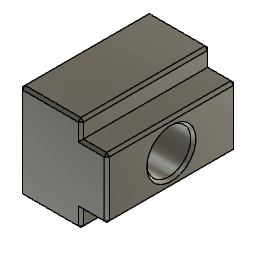
T-Nut_v0.1 (Autodesk Fusion 360 design; units mm, degrees)
Autodesk Fusion 360 part; units mm, degrees
sketch "Sketch1" plane through (0, 0, 0) normal (0, 1, 0) x (1, 0, 0)
  line L0 (-18.22, -14.04) -> (0, -14.04)
  line L1 (0, -14.04) -> (0, 14.04)
  line L2 (0, 14.04) -> (-18.22, 14.04)
  line L3 (-18.22, 14.04) -> (-18.22, -14.04)
  line L4 (0, -5.075) -> (-4, -5.075)
  line L5 (-4, -5.075) -> (-4, -7.75)
  line L6 (-4, -7.75) -> (-14.22, -7.75)
  line L7 (0, 5.075) -> (-4, 5.075)
  line L8 (-4, 5.075) -> (-4, 7.75)
  line L9 (-4, 7.75) -> (-14.22, 7.75)
  line L10 (-14.22, 7.75) -> (-14.22, -7.75)
  line L11 (-18.22, 0) -> (0, 0) construction
  line L12 (-4, -5.075) -> (-4, 5.075) construction
  point P0 (-14.22, 0)
  point P1 (-4, 0)
  dimension "d1" = 28.08
  dimension "d2" = 10.15
  dimension "d3" = 4
  dimension "d4" = 10.22
  dimension "d5" = 15.5
  dimension "d6" = 2.675
  dimension "d7" = 14.22
  dimension "d10" = 4
  constraint horizontal L0
  constraint vertical L1
  constraint horizontal L2
  constraint vertical L3
  constraint midpoint L11.end L1
  constraint coincident L1 L4.start
  constraint perpendicular L1 L4
  constraint perpendicular L4 L5
  constraint perpendicular L5 L6
  constraint coincident L1 L7.start
  constraint perpendicular L5 L7
  constraint perpendicular L7 L8
  constraint perpendicular L5 L9
  constraint perpendicular L6 L10
  constraint midpoint L3 L11.start
  constraint coincident L11.end origin
  constraint perpendicular L7 L12
  constraint midpoint L10 P0
  constraint coincident L11 P0
  constraint midpoint L12 P1
  constraint coincident L11 P1
  measures "d1" distance of L0 L2
  measures "d2" distance of L4 L7
  measures "d3" distance of L1 L5
  measures "d4" distance of L5 L10
  measures "d5" distance of L6 L9
  measures "d6" distance of L7 L9
  measures "d7" distance of L1 L10
  measures "d10" distance of L3 L10
extrude "Extrude1" add sketch "Sketch1" along normal blind 100 contours L0 L1 L2 L3 L4 L5 L6 L7 L8 L9 L10 makes body 1
sketch "Sketch2" plane through (0, 0, 0) normal (0, 1, 0) x (1, 0, 0)
  line L0 (-4, -7.75) -> (-14.22, -7.75)
  line L1 (-14.22, 7.75) -> (-14.22, -7.75)
  line L2 (-4, 7.75) -> (-14.22, 7.75)
  line L3 (-4, 5.075) -> (-4, 7.75)
  line L4 (0, 5.075) -> (-4, 5.075)
  line L5 (0, -5.075) -> (-4, -5.075)
  line L6 (-4, -5.075) -> (-4, -7.75)
  line L7 (0, -14.04) -> (0, 14.04)
  line L8 (0, 5.075) -> (0, -5.075)
  line L9 (-0.4, -4.675) -> (-4.4, -4.675)
  line L10 (-4.4, -4.675) -> (-4.4, -7.35)
  line L11 (-4.4, -7.35) -> (-13.82, -7.35)
  line L12 (-13.82, 7.35) -> (-13.82, -7.35)
  line L13 (-4.4, 7.35) -> (-13.82, 7.35)
  line L14 (-4.4, 4.675) -> (-4.4, 7.35)
  line L15 (-0.4, 4.675) -> (-4.4, 4.675)
  line L16 (-0.4, 4.675) -> (-0.4, -4.675)
  dimension "d11" = 0.4
  constraint coincident L4.start L8.start
  constraint coincident L5.start L8.end
extrude "Extrude2" add sketch "Sketch2" along normal mid plane 20 separate body contours L9 L10 L11 L12 L13 L14 L15 L16 makes body 2
sketch "Sketch4" plane through (-13.82, 0, 0) normal (-1, 0, 0) x (0, -1, 0)
  line L0 (10, 7.35) -> (-10, 7.35)
  line L1 (-10, 7.35) -> (-10, -7.35)
  line L2 (-10, -7.35) -> (10, -7.35)
  line L3 (10, -7.35) -> (10, 7.35)
  line L4 (3.3811, 5.8563) -> (-3.3811, 5.8562)
  line L5 (-3.3811, 5.8562) -> (-6.7622, 0)
  line L6 (-6.7622, 0) -> (-3.3811, -5.8563)
  line L7 (-3.3811, -5.8563) -> (3.3811, -5.8563)
  line L8 (3.3811, -5.8563) -> (6.7622, 0)
  line L9 (6.7622, 0) -> (3.3811, 5.8563)
  line L10 (0, 0) -> (10, 0) construction
  circle A0 centre (0, 0) radius 3.378
  dimension "d14" = 11.7125
  dimension "d23" = 6.756
  constraint coincident L10.start A0.centre
  constraint midpoint L3 L10.end
  measures "d14" distance of L4 L7
  measures "d23" diameter of A0
extrude "Extrude3" cut sketch "Sketch4" against normal blind 6.5563 contours L4 L5 L6 L7 L8 L9 bodies 2
extrude "Extrude4" cut sketch "Sketch4" against normal blind 25.66 contours A0 bodies 2
chamfer "Chamfer1" distance 0.4 angle 45 23 edges at (-9.11, 10, 7.35) (-4.4, 0, 7.35) (-9.11, -10, 7.35) (-4.4, 10, 6.0125) (-2.4, 10, 4.675) (-0.4, 10, 0) (-2.4, 10, -4.675) (-4.4, 10, -6.0125) (-9.11, 10, -7.35) (-4.4, 0, -7.35) (-4.4, -10, 6.0125) (-2.4, -10, 4.675) (-0.4, -10, 0) (-2.4, -10, -4.675) (-4.4, -10, -6.0125) (-9.11, -10, -7.35) (-0.4, 0, 4.675) (-0.4, 0, -4.675) (-0.4, 3.1494, -1.2215) (-13.82, 0, 7.35) (-13.82, -10, 0) (-13.82, 0, -7.35) (-13.82, 10, 0) on bodies 2
chamfer "Chamfer2" distance 0.4 angle 45 6 edges at (-13.82, 5.0717, 2.9281) (-13.82, 0, 5.8563) (-13.82, -5.0717, 2.9281) (-13.82, -5.0717, -2.9281) (-13.82, 0, -5.8563) (-13.82, 5.0717, -2.9281) on bodies 2
sketch "Sketch5" plane through (-7.2638, 0, 0) normal (-1, 0, 0) x (0, -1, 0)
  circle A0 centre (0, 0) radius 3.378
  line L0 (6.7622, 0) -> (3.3811, 5.8563)
  line L1 (3.3811, 5.8563) -> (-3.3811, 5.8562)
  line L2 (-3.3811, 5.8562) -> (-6.7622, 0)
  line L3 (-6.7622, 0) -> (-3.3811, -5.8563)
  line L4 (-3.3811, -5.8563) -> (3.3811, -5.8563)
  line L5 (3.3811, -5.8563) -> (6.7622, 0)
extrude "Extrude5" add sketch "Sketch5" against normal blind 0.2 contours A0 bodies 2
hidden bodies 1
equation "d14 = 7 in / 16 + 0.6 mm"
equation "d15 = -7 in / 32 - 1 mm"
named bodies: "T-nut"
